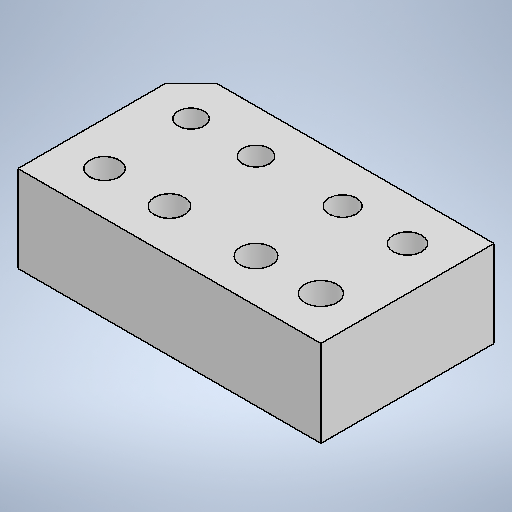
# Autodesk Inventor part: hole_test
Saved by Autodesk Inventor 2026.3 (Build 303398000, 398)
## iProperties
Created: 2026-06-10
Part Number: hole_test
Material: Generic
Document SubType Name: Modeling
Designer: gakut
Density: 1 g/cm^3
Appearance: Default
Author: gakut
## iProperties of the stored document hole_test_3DPrint.ipt
Created: 2026-06-10
Part Number: hole_test_3DPrint
Material: Generic
Document SubType Name: Modeling
Designer: gakut
Density: 1 g/cm^3
Appearance: Default
Author: gakut
Autodesk Inventor part; units mm, degrees
ref_plane "YZ Plane" through (0, 0, 0) normal (1, 0, 0) x (0, 1, 0)
ref_plane "XZ Plane" through (0, 0, 0) normal (0, 1, 0) x (-1, 0, 0)
ref_plane "XY Plane" through (0, 0, 0) normal (0, 0, 1) x (1, 0, 0)
sketch "Sketch1" plane through (0, 0, 0) normal (0, 1, 0) x (-1, 0, 0)
  line L0 (17.5, 10) -> (-17.5, 10)
  line L1 (-17.5, 10) -> (-17.5, -10)
  line L2 (-17.5, -10) -> (17.5, -10)
  line L3 (17.5, -10) -> (17.5, 10)
  line L4 (17.5, 10) -> (-17.5, -10) construction
  line L5 (-17.5, 10) -> (17.5, -10) construction
  circle A0 centre (12.5, -5) radius 1.5
  circle A1 centre (5, -5) radius 1.55
  circle A2 centre (-5, -5) radius 1.6
  circle A3 centre (-12.5, -5) radius 1.65
  circle A4 centre (12.5, 5) radius 1.7
  circle A5 centre (5, 5) radius 1.75
  circle A6 centre (-5, 5) radius 1.8
  circle A7 centre (-12.5, 5) radius 1.85
  line L6 (-5, 5) -> (5, 5)
  line L7 (5, 5) -> (5, -5)
  line L8 (5, -5) -> (-5, -5)
  line L9 (-5, -5) -> (-5, 5)
  line L10 (-5, 5) -> (5, -5) construction
  line L11 (5, 5) -> (-5, -5) construction
  line L12 (-12.5, 5) -> (12.5, 5)
  line L13 (12.5, 5) -> (12.5, -5)
  line L14 (12.5, -5) -> (-12.5, -5)
  line L15 (-12.5, -5) -> (-12.5, 5)
  line L16 (-12.5, 5) -> (12.5, -5) construction
  line L17 (12.5, 5) -> (-12.5, -5) construction
  point P0 (0, 0)
  dimension "d0" = 20
  dimension "d1" = 3
  dimension "d2" = 3.1
  dimension "d3" = 3.2
  dimension "d4" = 3.3
  dimension "d5" = 3.4
  dimension "d6" = 3.5
  dimension "d7" = 3.6
  dimension "d8" = 3.7
  dimension "d9" = 5
  dimension "d10" = 5
  dimension "d11" = 12.5
  dimension "d12" = 5
  constraints: 36 end point, 8 centre point, 8 coincident, 6 midpoint, 6 parallel, 3 horizontal, 3 perpendicular, 1 horizontal alignment, 1 point on line
  measures "d0" distance of L0.end L1.end
  measures "d1" diameter of A0
  measures "d2" diameter of A1
  measures "d3" diameter of A2
  measures "d4" diameter of A3
  measures "d5" diameter of A4
  measures "d6" diameter of A5
  measures "d7" diameter of A6
  measures "d8" diameter of A7
  measures "d9" distance from line of point (0, 0) L14
  measures "d10" distance from line of L9 point (0, 0)
  measures "d11" distance from line of L15 point (0, 0)
  measures "d12" distance from line of L1 A3.centre
extrude "Extrusion1" add sketch "Sketch1" along normal blind 10 contours L3 L2 L1 L0 | A0 L14 A1 L7 A5 L12 A4 L13 | A1 L8 A2 L9 A6 L6 A5 L7 | A2 L14 A3 L15 A7 L12 A6 L9
chamfer "Chamfer1" distance 3 angle 45 1 edges at (-17.5, 5, -10)
equation "\"d9\" = 0.25 * d0"
equation "\"d11\" = 2.5 * d10"
equation "\"d12\" = d9"
body "Solid1"
